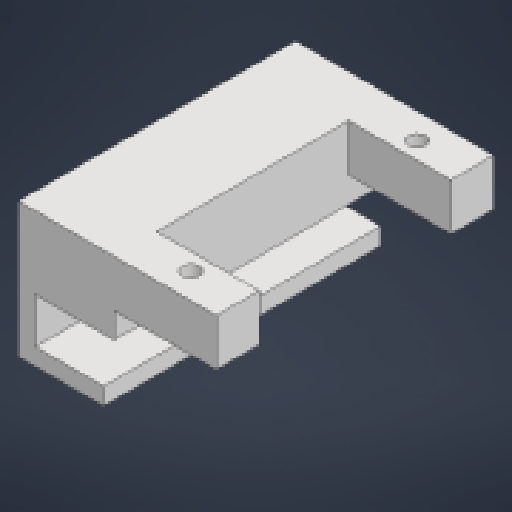
# Autodesk Inventor part: obj_3_外1壳.STL
Saved by Autodesk Inventor 2025 (Build 290162000, 162)
## iProperties
Created: 2026-04-25
Part Number: obj_3_外1壳.STL
Material: 常规
Document SubType Name: Modeling
Designer: XH
Density: 1 g/cm^3
Appearance: 默认
Author: XH
Autodesk Inventor part; units mm, degrees
ref_plane "YZ Plane" through (0, 0, 0) normal (1, 0, 0) x (0, 1, 0)
ref_plane "XZ Plane" through (0, 0, 0) normal (0, 1, 0) x (-1, 0, 0)
ref_plane "XY Plane" through (0, 0, 0) normal (0, 0, 1) x (1, 0, 0)
sketch "草图2" plane through (0, 0, 0) normal (0, 0, 1) x (1, 0, 0)
  line L0 (149.1878, 129.8039) -> (177.4063, 129.8039) projected
  line L1 (177.4063, 129.8039) -> (177.4063, 124.3039) projected
  line L2 (177.4063, 124.3039) -> (165.4062, 124.3039) projected
  line L3 (165.4062, 124.3039) -> (165.4062, 121.3039) projected
  line L4 (165.4062, 121.3039) -> (151.1878, 121.3039) projected
  line L5 (151.1878, 116.0039) -> (159.1878, 116.0039) projected
  line L6 (151.1878, 121.3039) -> (151.1878, 116.0039) projected
  line L7 (159.1878, 116.0039) -> (159.1878, 114.0039) projected
  line L8 (159.1878, 114.0039) -> (149.1878, 114.0039) projected
  line L9 (149.1878, 114.0039) -> (149.1878, 129.8039) projected
  point P0 (0, 0)
extrude "拉伸1" add sketch "草图2" along normal blind 32.5
sketch "草图3" plane through (165.4062, 124.3039, 0) normal (0, -1, 0) x (1, 0, 0)
  line L0 (0, 0) -> (0, 32.5) projected
  line L1 (12, 0) -> (12, 32.5) projected
  line L2 (0, 27.4986) -> (12, 27.4986)
  line L3 (12, 27.4986) -> (12, 4.9993)
  line L4 (12, 4.9993) -> (0, 4.9993)
  line L5 (0, 4.9993) -> (0, 27.4986)
  point P0 (-165.4062, 0)
  constraints: 8 end point, 2 parallel, 2 point on line, 1 horizontal, 1 perpendicular
extrude "拉伸2" cut sketch "草图3" against normal blind 24.5
sketch "草图4" plane through (165.4062, 124.3039, 32.5) normal (0, -1, 0) x (1, 0, 0)
  circle A0 centre (5.9961, -3.0044) radius 1
  point P0 (-165.4062, -32.5)
  dimension "d4" = 2
  constraints: 1 centre point
  measures "d4" diameter of A0
extrude "拉伸3" cut sketch "草图4" against normal blind 24.5
ref_plane "工作平面1" through (0, 0, 16.25) normal (0, 0, 1) x (1, 0, 0)
mirror "镜像1" about plane through (0, 0, 16.25) normal (0, 0, 1) of "拉伸3"
move faces "移动1" translate (5, 0, 0) faces at (151.1878, 117.7705, 10.8333) (159.1878, 114.6705, 10.8333) (149.1878, 124.5372, 10.8333)
sketch "草图5" plane through (154.1878, 114.0039, 0) normal (-1, 0, 0) x (0, 0, 1)
  circle A0 centre (8.302, 7.8986) radius 1.55 projected
  circle A1 centre (22.639, 7.8986) radius 1.55 projected
  circle A2 centre (8.302, 7.8986) radius 2.55
  circle A3 centre (22.639, 7.8986) radius 2.55
  point P0 (0, -114.0039)
  dimension "d12" = 1
  dimension "d13" = 1
  constraints: 2 centre point
  measures "d12" radial gap between concentric circles of A0 A2
  measures "d13" radial gap between concentric circles of A1 A3
extrude "拉伸4" cut sketch "草图5" against normal up to surface (2 mm away) contours A0 | A1
